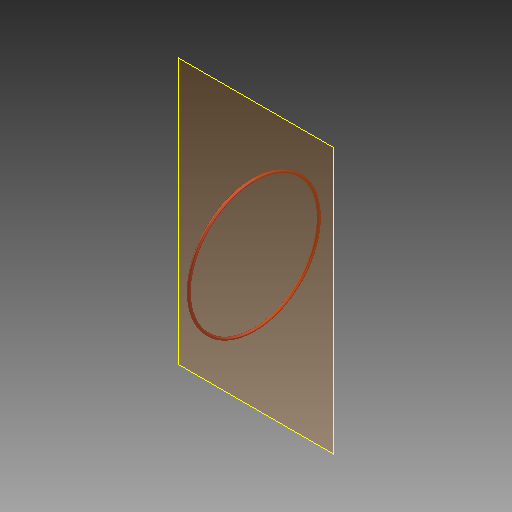
# Autodesk Inventor part: wheel_ring
Saved by Autodesk Inventor 2020 (Build 240168000, 168)
## iProperties
Created: 2024-10-05
Part Number: wheel_ring
Material: Типовые
Document SubType Name: Modeling
Designer: Ivan
Density: 1 g/cm^3
Appearance: Медь — сатинированная
Author: Ivan
Autodesk Inventor part; units mm, degrees
ref_plane "YZ Plane" through (0, 0, 0) normal (1, 0, 0) x (0, 1, 0)
ref_plane "XZ Plane" through (0, 0, 0) normal (0, 1, 0) x (-1, 0, 0)
ref_plane "XY Plane" through (0, 0, 0) normal (0, 0, 1) x (1, 0, 0)
ref_plane "РабПлоскость1" through (-3, 0, 0) normal (0, 0, 1) x (1, 0, 0)
sketch "Эскиз1" plane through (-3, 0, 0) normal (0, 0, 1) x (1, 0, 0)
  line L0 (0.75, 46.2499) -> (0.75, 1.2499)
  line L1 (0.75, 1.2499) -> (0, 1.2499)
  line L2 (0, 0.75) -> (0, 0.1136)
  line L3 (0, 0.75) -> (0, 2.3824)
  circle A0 centre (0, 1.2499) radius 0.5
  line L4 (31.8636, 21.7045) -> (-30.4999, 21.7045)
  line L5 (35.0499, 23.7499) -> (-33.5499, 23.7499)
  point P0 (3, 0)
  dimension "d0" = 1
  constraints: 12 end point, 2 horizontal, 2 vertical, 1 centre point, 1 coincident, 1 point on line, 5 other
  measures "d0" diameter of A0
revolve "Вращение1" add sketch "Эскиз1" angle 360 about axis through (32.0499, 23.7499, 0) along (-1, 0, 0)
